Autodesk Inventor part; units mm, degrees
(part 2 of 2)
  arc A357 (20.6705, 39.2812) -> (21.9493, 39.6313) centre (21.1348, 40.0956) ccw
  arc A358 (22.9266, 39.074) -> (23.2766, 37.7952) centre (23.741, 38.6097) ccw
  line L359 (22.2221, 39.7059) -> (22.8519, 39.3468)
  arc A359 (22.2221, 39.7059) -> (21.9493, 39.6313) centre (22.123, 39.5322) ccw
  arc A360 (22.9266, 39.074) -> (22.8519, 39.3468) centre (22.7528, 39.1731) ccw
  line L360 (19.9312, 40.9023) -> (20.257, 40.7435)
  line L361 (20.257, 40.7435) -> (19.6053, 41.0611)
  line L362 (19.6053, 41.0611) -> (20.257, 40.7435)
  arc A361 (18.0845, 40.5368) -> (19.3379, 40.9689) centre (18.4951, 41.3796) ccw
  arc A362 (20.3492, 40.4761) -> (20.7813, 39.2227) centre (21.192, 40.0654) ccw
  line L363 (19.6053, 41.0611) -> (20.257, 40.7435)
  arc A363 (19.6053, 41.0611) -> (19.3379, 40.9689) centre (19.5177, 40.8813) ccw
  arc A364 (20.3492, 40.4761) -> (20.257, 40.7435) centre (20.1694, 40.5637) ccw
  line L364 (17.2418, 42.1067) -> (17.5772, 41.9693)
  line L365 (17.5772, 41.9693) -> (16.9063, 42.244)
  line L366 (16.9063, 42.244) -> (17.5772, 41.9693)
  arc A365 (15.4226, 41.6224) -> (16.6454, 42.1347) centre (15.7779, 42.49) ccw
  arc A366 (17.6865, 41.7084) -> (18.1989, 40.4856) centre (18.5541, 41.3532) ccw
  line L367 (16.9063, 42.244) -> (17.5772, 41.9693)
  arc A367 (16.9063, 42.244) -> (16.6454, 42.1347) centre (16.8305, 42.0589) ccw
  arc A368 (17.6865, 41.7084) -> (17.5772, 41.9693) centre (17.5014, 41.7842) ccw
  line L368 (14.4801, 43.1344) -> (14.8237, 43.0191)
  line L369 (14.8237, 43.0191) -> (14.1364, 43.2498)
  line L370 (14.1364, 43.2498) -> (14.8237, 43.0191)
  arc A369 (12.696, 42.5334) -> (13.8832, 43.1238) centre (12.9944, 43.4222) ccw
  arc A370 (14.9497, 42.7658) -> (15.5401, 41.5787) centre (15.8384, 42.4675) ccw
  line L371 (14.1364, 43.2498) -> (14.8237, 43.0191)
  arc A371 (14.1364, 43.2498) -> (13.8832, 43.1238) centre (14.0728, 43.0602) ccw
  arc A372 (14.9497, 42.7658) -> (14.8237, 43.0191) centre (14.7601, 42.8295) ccw
  line L372 (11.6576, 43.9812) -> (12.008, 43.8884)
  line L373 (12.008, 43.8884) -> (11.3072, 44.0741)
  line L374 (11.3072, 44.0741) -> (12.008, 43.8884)
  arc A373 (9.9162, 43.266) -> (11.0626, 43.932) centre (10.1564, 44.1722) ccw
  arc A374 (12.1501, 43.6438) -> (12.8161, 42.4974) centre (13.0563, 43.4036) ccw
  line L375 (11.3072, 44.0741) -> (12.008, 43.8884)
  arc A375 (11.3072, 44.0741) -> (11.0626, 43.932) centre (11.256, 43.8808) ccw
  arc A376 (12.1501, 43.6438) -> (12.008, 43.8884) centre (11.9568, 43.695) ccw
  line L376 (8.7863, 44.6436) -> (9.1419, 44.5736)
  line L377 (9.1419, 44.5736) -> (8.4306, 44.7136)
  line L378 (8.4306, 44.7136) -> (9.1419, 44.5736)
  arc A377 (7.0948, 43.8172) -> (8.1957, 44.556) centre (7.2759, 44.737) ccw
  arc A378 (9.2996, 44.3388) -> (10.0384, 43.2379) centre (10.2194, 44.1577) ccw
  line L379 (8.4306, 44.7136) -> (9.1419, 44.5736)
  arc A379 (8.4306, 44.7136) -> (8.1957, 44.556) centre (8.392, 44.5174) ccw
  arc A380 (9.2996, 44.3388) -> (9.1419, 44.5736) centre (9.1033, 44.3774) ccw
  line L380 (5.8781, 45.1187) -> (6.2375, 45.0719)
  line L381 (6.2375, 45.0719) -> (5.5186, 45.1655)
  line L382 (5.5186, 45.1655) -> (6.2375, 45.0719)
  arc A381 (4.2437, 44.1845) -> (5.2944, 44.9931) centre (4.3648, 45.1142) ccw
  arc A382 (6.41, 44.8477) -> (7.2185, 43.797) centre (7.3397, 44.7266) ccw
  line L383 (5.5186, 45.1655) -> (6.2375, 45.0719)
  arc A383 (5.5186, 45.1655) -> (5.2944, 44.9931) centre (5.4928, 44.9672) ccw
  arc A384 (6.41, 44.8477) -> (6.2375, 45.0719) centre (6.2117, 44.8736) ccw
  line L384 (2.9452, 45.4046) -> (3.3069, 45.3811)
  line L385 (3.3069, 45.3811) -> (2.5835, 45.428)
  line L386 (2.5835, 45.428) -> (3.3069, 45.3811)
  arc A385 (1.3747, 44.3666) -> (2.3709, 45.2414) centre (1.4354, 45.3021) ccw
  arc A386 (3.4936, 45.1686) -> (4.3684, 44.1724) centre (4.4291, 45.1079) ccw
  line L387 (2.5835, 45.428) -> (3.3069, 45.3811)
  arc A387 (2.5835, 45.428) -> (2.3709, 45.2414) centre (2.5705, 45.2285) ccw
  arc A388 (3.4936, 45.1686) -> (3.3069, 45.3811) centre (3.294, 45.1815) ccw
  point P0 (3.3325, 45.3778)
  point P1 (2.5577, 45.4281)
  point P2 (1.4374, 44.3646)
  point P3 (0.3882, 45.4983)
  point P4 (-0.3882, 45.4983)
  point P5 (-1.4374, 44.3646)
  point P6 (-2.5577, 45.4281)
  point P7 (-3.3325, 45.3778)
  point P8 (-4.3061, 44.1785)
  point P9 (-5.4929, 45.1672)
  point P10 (-6.2628, 45.0669)
  point P11 (-7.1567, 43.8071)
  point P12 (-8.4051, 44.7169)
  point P13 (-9.1668, 44.567)
  point P14 (-9.9773, 43.252)
  point P15 (-11.282, 44.0791)
  point P16 (-12.0324, 43.8802)
  point P17 (-12.7561, 42.5155)
  point P18 (-14.1115, 43.2564)
  point P19 (-14.8475, 43.0093)
  point P20 (-15.4814, 41.6006)
  point P21 (-16.8819, 42.2522)
  point P22 (-17.6004, 41.958)
  point P23 (-18.1417, 40.5113)
  point P24 (-19.5815, 41.0709)
  point P25 (-20.2794, 40.7308)
  point P26 (-20.7259, 39.252)
  point P27 (-22.1989, 39.7172)
  point P28 (-22.8734, 39.3327)
  point P29 (-23.2232, 37.8281)
  point P30 (-24.7233, 38.197)
  point P31 (-25.3714, 37.7696)
  point P32 (-25.6231, 36.2455)
  point P33 (-27.1439, 36.5166)
  point P34 (-27.763, 36.0481)
  point P35 (-27.9156, 34.5109)
  point P36 (-29.4507, 34.683)
  point P37 (-30.0382, 34.1754)
  point P38 (-30.0909, 32.6316)
  point P39 (-31.6339, 32.7039)
  point P40 (-32.1873, 32.1594)
  point P41 (-32.14, 30.6154)
  point P42 (-33.6845, 30.5876)
  point P43 (-34.2015, 30.0084)
  point P44 (-34.0544, 28.4707)
  point P45 (-35.5938, 28.3431)
  point P46 (-36.0722, 27.7317)
  point P47 (-35.8259, 26.2067)
  point P48 (-37.3538, 25.9797)
  point P49 (-37.7916, 25.3385)
  point P50 (-37.4471, 23.8327)
  point P51 (-38.9571, 23.5073)
  point P52 (-39.3525, 22.8392)
  point P53 (-38.9112, 21.3588)
  point P54 (-40.397, 20.9363)
  point P55 (-40.7484, 20.244)
  point P56 (-40.2122, 18.7953)
  point P57 (-41.6675, 18.2775)
  point P58 (-41.9733, 17.5639)
  point P59 (-41.3445, 16.153)
  point P60 (-42.7632, 15.542)
  point P61 (-43.0222, 14.8101)
  point P62 (-42.3033, 13.4429)
  point P63 (-43.6796, 12.7414)
  point P64 (-43.8906, 11.9943)
  point P65 (-43.0848, 10.6764)
  point P66 (-44.4127, 9.8873)
  point P67 (-44.575, 9.1281)
  point P68 (-43.6855, 7.8651)
  point P69 (-44.9596, 6.9917)
  point P70 (-45.0724, 6.2236)
  point P71 (-44.103, 5.0209)
  point P72 (-45.3179, 4.0668)
  point P73 (-45.3807, 3.293)
  point P74 (-44.3355, 2.1556)
  point P75 (-45.4861, 1.1249)
  point P76 (-45.4987, 0.3486)
  point P77 (-44.3821, -0.7188)
  point P78 (-45.4635, -1.8218)
  point P79 (-45.4258, -2.5972)
  point P80 (-44.2425, -3.5901)
  point P81 (-45.2502, -4.7608)
  point P82 (-45.1624, -5.5322)
  point P83 (-43.9173, -6.4464)
  point P84 (-44.8472, -7.6799)
  point P85 (-44.7096, -8.4439)
  point P86 (-43.4079, -9.2756)
  point P87 (-44.256, -10.5667)
  point P88 (-44.0693, -11.3203)
  point P89 (-42.7165, -12.066)
  point P90 (-43.4792, -13.4092)
  point P91 (-43.2441, -14.1491)
  point P92 (-41.8458, -14.8057)
  point P93 (-42.5201, -16.1955)
  point P94 (-42.2375, -16.9186)
  point P95 (-40.7997, -17.4833)
  point P96 (-41.3826, -18.9139)
  point P97 (-41.0538, -19.6172)
  point P98 (-39.5825, -20.0876)
  point P99 (-40.0715, -21.5529)
  point P100 (-39.6979, -22.2335)
  point P101 (-38.1992, -22.6076)
  point P102 (-38.5923, -24.1015)
  point P103 (-38.1755, -24.7565)
  point P104 (-36.6557, -25.0329)
  point P105 (-36.9513, -26.549)
  point P106 (-36.4929, -27.1756)
  point P107 (-34.9584, -27.3531)
  point P108 (-35.1553, -28.8852)
  point P109 (-34.6573, -29.4808)
  point P110 (-33.1146, -29.5586)
  point P111 (-33.2118, -31.1002)
  point P112 (-32.6764, -31.6624)
  point P113 (-31.1318, -31.6401)
  point P114 (-31.1291, -33.1848)
  point P115 (-30.5583, -33.7111)
  point P116 (-29.0185, -33.5889)
  point P117 (-28.9158, -35.1302)
  point P118 (-28.3121, -35.6184)
  point P119 (-26.7834, -35.3968)
  point P120 (-26.5811, -36.9282)
  point P121 (-25.9472, -37.3764)
  point P122 (-24.436, -37.0562)
  point P123 (-24.135, -38.5714)
  point P124 (-23.4734, -38.9775)
  point P125 (-21.9861, -38.5603)
  point P126 (-21.5877, -40.0527)
  point P127 (-20.9012, -40.4152)
  point P128 (-19.444, -39.9026)
  point P129 (-18.9498, -41.3661)
  point P130 (-18.2413, -41.6834)
  point P131 (-16.8203, -41.0775)
  point P132 (-16.2325, -42.506)
  point P133 (-15.5049, -42.7767)
  point P134 (-14.1261, -42.0801)
  point P135 (-13.447, -43.4675)
  point P136 (-12.7034, -43.6907)
  point P137 (-11.3727, -42.9062)
  point P138 (-10.6052, -44.2468)
  point P139 (-9.8487, -44.4213)
  point P140 (-8.5715, -43.5524)
  point P141 (-7.7188, -44.8405)
  point P142 (-6.9526, -44.9657)
  point P143 (-5.7344, -44.0159)
  point P144 (-4.8001, -45.2461)
  point P145 (-4.0274, -45.3214)
  point P146 (-2.8732, -44.2948)
  point P147 (-1.8613, -45.4619)
  point P148 (-1.0853, -45.4871)
  point P149 (0, -44.3879)
  point P150 (1.0853, -45.4871)
  point P151 (1.8613, -45.4619)
  point P152 (2.8732, -44.2948)
  point P153 (4.0274, -45.3214)
  point P154 (4.8001, -45.2461)
  point P155 (5.7344, -44.0159)
  point P156 (6.9526, -44.9657)
  point P157 (7.7188, -44.8405)
  point P158 (8.5715, -43.5524)
  point P159 (9.8487, -44.4213)
  point P160 (10.6052, -44.2468)
  point P161 (11.3727, -42.9062)
  point P162 (12.7034, -43.6907)
  point P163 (13.447, -43.4675)
  point P164 (14.1261, -42.0801)
  point P165 (15.5049, -42.7767)
  point P166 (16.2325, -42.506)
  point P167 (16.8203, -41.0775)
  point P168 (18.2413, -41.6834)
  point P169 (18.9498, -41.3661)
  point P170 (19.444, -39.9026)
  point P171 (20.9012, -40.4152)
  point P172 (21.5877, -40.0527)
  point P173 (21.9861, -38.5603)
  point P174 (23.4734, -38.9775)
  point P175 (24.135, -38.5714)
  point P176 (24.436, -37.0562)
  point P177 (25.9472, -37.3764)
  point P178 (26.5811, -36.9282)
  point P179 (26.7834, -35.3968)
  point P180 (28.3121, -35.6184)
  point P181 (28.9158, -35.1302)
  point P182 (29.0185, -33.5889)
  point P183 (30.5583, -33.7111)
  point P184 (31.1291, -33.1848)
  point P185 (31.1318, -31.6401)
  point P186 (32.6764, -31.6624)
  point P187 (33.2118, -31.1002)
  point P188 (33.1146, -29.5586)
  point P189 (34.6573, -29.4808)
  point P190 (35.1553, -28.8852)
  point P191 (34.9584, -27.3531)
  point P192 (36.4929, -27.1756)
  point P193 (36.9513, -26.549)
  point P194 (36.6557, -25.0329)
  point P195 (38.1755, -24.7565)
  point P196 (38.5923, -24.1015)
  point P197 (38.1992, -22.6076)
  point P198 (39.6979, -22.2335)
  point P199 (40.0715, -21.5529)
  dimension "d24" = 360
  constraints: 776 end point, 776 point on circle, 388 centre point, 4 horizontal, 1 coincident, 1846 other
extrude "Extrusion2" add sketch "Sketch2" along normal blind 12 contours A296 A294 A289 A291 A0 A292 A290 A285 A287 A288 A286 A281 A283 A284 A282 A277 A279 A280 A278 A273 A275 A276 A274 A269 A271 A272 A270 A265 A267 A268 A266 A261 A263 A264 A262 A257 A259 A260 A258 A253 A255 A256 A254 A249 A251 A252 A250 A245 A247 A248 A246 A241 A243 A244 A242 A237 A239 A240 A238 A233 A235 A236 A234 A229 A231 A232 A230 A225 A227 A228 A226 A221 A223 A224 A222 A217 A219 A220 A218 A213 A215 A216 A214 A209 A211 A212 A210 A205 A207 A208 A206 A201 A203 A204 A202 A197 A199 A200 A198 A193 A195 A196 A194 A189 A191 A192 A190 A185 A187 A188 A186 A181 A183 A184 A182 A177 A179 A180 A178 A173 A175 A176 A174 A169 A171 A172 A170 A165 A167 A168 A166 A161 A163 A164 A162 A157 A159 A160 A158 A153 A155 A156 A154 A149 A151 A152 A150 A145 A147 A148 A146 A141 A143 A144 A142 A137 A139 A140 A138 A133 A135 A136 A134 A129 A131 A132 A130 A125 A127 A128 A126 A121 A123 A124 A122 A117 A119 A120 A118 A113 A115 A116 A114 A109 A111 A112 A110 A105 A107 A108 A106 A101 A103 A104 A102 A97 A99 A100 A98 A93 A95 A96 A94 A89 A91 A92 A90 A85 A87 A88 A86 A81 A83 A84 A82 A77 A79 A80 A78 A73 A75 A76 A74 A69 A71 A72 A70 A65 A67 A68 A66 A61 A63 A64 A62 A57 A59 A60 A58 A53 A55 A56 A54 A49 A51 A52 A50 A45 A47 A48 A46 A41 A43 A44 A42 A37 A39 A40 A38 A33 A35 A36 A34 A29 A31 A32 A30 A25 A27 A28 A26 A21 A23 A24 A22 A17 A19 A20 A18 A13 A15 A16 A14 A9 A11 A12 A10 A5 A7 A8 A6 A1 A3 A4 A2 A385 A387 A388 A386 A381 A383 A384 A382 A377 A379 A380 A378 A373 A375 A376 A374 A369 A371 A372 A370 A365 A367 A368 A366 A361 A363 A364 A362 A357 A359 A360 A358 A353 A355 A356 A354 A349 A351 A352 A350 A345 A347 A348 A346 A341 A343 A344 A342 A337 A339 A340 A338 A333 A335 A336 A334 A329 A331 A332 A330 A325 A327 A328 A326 A321 A323 A324 A322 A317 A319 A320 A318 A313 A315 A316 A314 A309 A311 A312 A310 A305 A307 A308 A306 A301 A303 A304 A302 A297 A299 A300 A298 A293 A295
sketch "Sketch3" plane through (0, 14, 0) normal (0, 1, 0) x (1, 0, 0)
  line L0 (2.5994, 26.7731) -> (2.5994, -25)
  line L1 (-26, 12) -> (-26, 8.9443)
  line L2 (-26, -8.9443) -> (-26, -12)
  line L3 (-24, 8.9443) -> (-24, 12)
  line L4 (-24, -12) -> (-24, -8.9443)
  line L5 (-24, 8.9443) -> (-24, 12)
  line L6 (-35.2416, 0) -> (31.0706, 0)
  circle A0 centre (0, 0) radius 25
  arc A1 (-26, 8.9443) -> (-26, -8.9443) centre (-25, 0) ccw
  arc A2 (-24, -8.9443) -> (-24, 8.9443) centre (-25, 0) ccw
  line L7 (25, 0) -> (25.7159, 0.8538)
  line L8 (0, -25) -> (0.4021, -24.3276)
  line L9 (-12, -26) -> (-8.9443, -26)
  line L10 (8.9443, -26) -> (12, -26)
  line L11 (-8.9443, -24) -> (-12, -24)
  line L12 (12, -24) -> (8.9443, -24)
  line L13 (-8.9443, -24) -> (-12, -24)
  arc A3 (-8.9443, -26) -> (8.9443, -26) centre (0, -25) ccw
  arc A4 (8.9443, -24) -> (-8.9443, -24) centre (0, -25) ccw
  line L14 (24, 12) -> (24, 8.9443)
  line L15 (24, -8.9443) -> (24, -12)
  line L16 (26, 8.9443) -> (26, 12)
  line L17 (26, -12) -> (26, -8.9443)
  line L18 (26, 8.9443) -> (26, 12)
  arc A5 (24, 8.9443) -> (24, -8.9443) centre (25, 0) ccw
  arc A6 (26, -8.9443) -> (26, 8.9443) centre (25, 0) ccw
  line L19 (-24, 12) -> (-24, 14)
  line L20 (-24, 14) -> (-26, 14)
  line L21 (-26, 14) -> (-26, 12)
  line L22 (-24, -12) -> (-24, -14)
  line L23 (-24, -14) -> (-26, -14)
  line L24 (-26, -14) -> (-26, -12)
  line L25 (26, 12) -> (26, 14)
  line L26 (26, 14) -> (24, 14)
  line L27 (24, 14) -> (24, 12)
  line L28 (26, -12) -> (26, -14)
  line L29 (26, -14) -> (24, -14)
  line L30 (24, -14) -> (24, -12)
  line L31 (12, -24) -> (14, -24)
  line L32 (14, -24) -> (14, -26)
  line L33 (14, -26) -> (12, -26)
  line L34 (-12, -24) -> (-14, -24)
  line L35 (-14, -24) -> (-14, -26)
  line L36 (-14, -26) -> (-12, -26)
  point P0 (14.7584, 0)
  constraints: 74 end point, 18 parallel, 14 point on circle, 7 centre point, 3 horizontal, 2 perpendicular, 1 coincident, 1 point on line, 1 vertical
extrude "Extrusion3" cut sketch "Sketch3" against normal through all contours A5 L14 L27 L26 L25 L16 A6 L17 L28 L29 L30 L15 A0 | A0 L6 A5 | A2 L6 A0 | A0 L6 A1 L1 L21 L20 L19 L3 A2 | A4 A0 L0 | L0 A0 A4 | A2 A0 L6 | L6 A0 A5 | A0 A2 L4 L22 L23 L24 L2 A1 L6 | A0 A4 L12 L31 L32 L33 L10 A3 L9 L36 L35 L34 L11
sketch "Sketch5" plane through (0, 0, 0) normal (0, -1, 0) x (1, 0, 0)
  circle A0 centre (0, 0) radius 14
  dimension "d46" = 28
  constraints: 1 centre point, 1 coincident
  measures "d46" diameter of A0
extrude "Extrusion4" cut sketch "Sketch5" against normal blind 10
sketch "Sketch6" plane through (0, 10, 0) normal (0, -1, 0) x (1, 0, 0)
  circle A0 centre (0, 0) radius 9
  dimension "d49" = 18
  constraints: 1 centre point, 1 coincident
  measures "d49" diameter of A0
extrude "Extrusion5" cut sketch "Sketch6" against normal through all
fillet "Fillet2" radius 1 12 edges at (-24, 7, -14) (-26, 7, -14) (-26, 7, 14) (-24, 7, 14) (-14, 7, 26) (-14, 7, 24) (14, 7, 26) (14, 7, 24) (26, 7, 14) (24, 7, 14) (24, 7, -14) (26, 7, -14)
body "Solid1"
